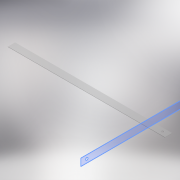
# Autodesk Inventor part: encoder-linear-strip
Saved by Autodesk Inventor 2016 (Build 200138000, 138)
## iProperties
Created: 2015-05-21
Part Number: encoder-linear-strip
Material: Polycarbonate, Clear
Document SubType Name: Modeling
Designer: as
Mass: 0.261858 g
Surface Area: 17.2729 cm^2
Volume: 0.218215 cm^3
Density: 1.2 g/cm^3
Appearance: Polycarbonate - Clear
Author: as
Autodesk Inventor part; units mm, degrees
ref_plane "YZ Plane" through (0, 0, 0) normal (1, 0, 0) x (0, 1, 0)
ref_plane "XZ Plane" through (0, 0, 0) normal (0, 1, 0) x (-1, 0, 0)
ref_plane "XY Plane" through (0, 0, 0) normal (0, 0, 1) x (1, 0, 0)
sketch "Sketch1" plane through (0, 0, 0) normal (0, 0, 1) x (1, 0, 0)
  line L0 (65, -3) -> (-65, -3)
  line L1 (-65, -3) -> (-65, 3)
  line L2 (-65, 3) -> (65, 3)
  line L3 (65, 3) -> (65, -3)
  line L4 (65, -3) -> (-65, 3) construction
  line L5 (-65, -3) -> (65, 3) construction
  point P0 (0, 0)
  dimension "d0" = 130
  dimension "d1" = 6
  constraints: 12 end point, 2 midpoint, 2 parallel, 1 horizontal, 1 perpendicular
  measures "d0" distance of L1.end L2.end
  measures "d1" distance of L0.end L1.end
extrude "Extrusion1" add sketch "Sketch1" along normal blind 0.25
sketch "Sketch2" plane through (0, 0, 0.25) normal (0, 0, 1) x (1, 0, 0)
  circle A0 centre (60, 0) radius 1
  point P0 (0, 0)
  dimension "d4" = 2
  constraints: 1 centre point
  measures "d4" diameter of A0
extrude "Extrusion2" cut sketch "Sketch2" against normal blind 0.25
sketch "Sketch4" plane through (0, 0, 0.25) normal (0, 0, 1) x (1, 0, 0)
  line L0 (51.75, -3) -> (52.25, -3)
  line L1 (52.25, -3) -> (52.25, 3)
  line L2 (52.25, 3) -> (51.75, 3)
  line L3 (51.75, 3) -> (51.75, -3)
  line L4 (51.75, -3) -> (52.25, 3) construction
  line L5 (52.25, -3) -> (51.75, 3) construction
  point P0 (0, 0)
  point P1 (52, 0)
  dimension "d18" = 0.5
  dimension "d19" = 6
  constraints: 12 end point, 2 midpoint, 2 parallel, 1 horizontal, 1 perpendicular
  measures "d18" distance of L2.end L1.end
  measures "d19" distance of L1.end L0.end
extrude "Extrusion3" add sketch "Sketch4" along normal blind 0.08
pattern_linear "Rectangular Pattern3" count 100 spacing 1 along (-1, 0, 0) of "Extrusion3"
body "Solid1"
